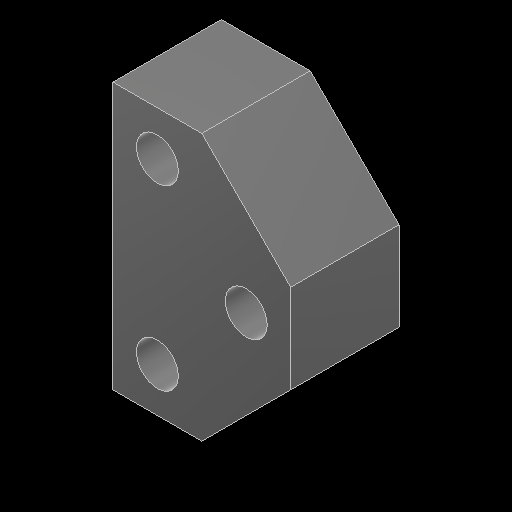
# Autodesk Inventor part: MiddleClampingTopPiece
Saved by Autodesk Inventor 2022 (Build 260153000, 153)
## iProperties
Created: 2022-06-15
Part Number: MiddleClampingTopPiece
Material: Custom TPU
Document SubType Name: Modeling
Designer: tandu
Density: 1.21 g/cm^3
Appearance: Smooth - Black
Mass: 1.40608 g
Surface Area: 10.8835 cm^2
Volume: 1.16205 cm^3
Author: tandu
Autodesk Inventor part; units mm, degrees
ref_plane "YZ Plane" through (0, 0, 0) normal (1, 0, 0) x (0, 1, 0)
ref_plane "XZ Plane" through (0, 0, 0) normal (0, 1, 0) x (-1, 0, 0)
ref_plane "XY Plane" through (0, 0, 0) normal (0, 0, 1) x (1, 0, 0)
sketch "Sketch1" plane through (0, 0, 0) normal (0, 0, 1) x (1, 0, 0)
  line L0 (5.85, -9.525) -> (-6.85, -9.525) projected
  line L1 (5.85, -9.525) -> (5.85, 9.525) projected
  line L2 (-6.85, 9.525) -> (5.85, 9.525) projected
  line L3 (-6.85, 3.175) -> (-6.85, 9.525) projected
  line L4 (-6.85, 3.175) -> (-0.5, 3.175) projected
  line L5 (-0.5, 3.175) -> (-0.5, -3.175) projected
  line L6 (-0.5, -3.175) -> (-6.85, -3.175) projected
  line L7 (-6.85, -9.525) -> (-6.85, -3.175) projected
  circle A0 centre (-3.675, -6.35) radius 1.5 projected
  circle A1 centre (2.675, 0) radius 1.5 projected
  circle A2 centre (-3.675, 6.35) radius 1.5 projected
  line L8 (-6.85, 3.175) -> (-6.85, -3.175)
  line L9 (-0.5, -9.525) -> (5.85, -3.175)
  line L10 (5.85, 3.175) -> (-0.5, 9.525)
  point P0 (0, 0)
  constraints: 6 end point, 2 horizontal alignment, 2 midpoint, 2 point on line, 1 vertical, 1 other
extrude "Extrusion1" add sketch "Sketch1" along normal blind 5.842 contours L0 L7 L6 L5 L4 L3 L2 L10 L1 L9
sketch "Sketch2" plane through (0, 0, 5.842) normal (0, 0, 1) x (1, 0, 0)
  line L0 (-6.85, 3.175) -> (-0.5, 3.175) projected
  line L1 (-0.5, 3.175) -> (-0.5, -3.175) projected
  line L2 (-0.5, -3.175) -> (-6.85, -3.175) projected
  line L3 (-6.85, -3.175) -> (-6.85, -9.525) projected
  line L4 (-6.85, -9.525) -> (-0.5, -9.525) projected
  line L5 (-0.5, -9.525) -> (5.85, -3.175) projected
  line L6 (5.85, -3.175) -> (5.85, 3.175) projected
  line L7 (5.85, 3.175) -> (-0.5, 9.525) projected
  line L8 (-0.5, 9.525) -> (-6.85, 9.525) projected
  line L9 (-6.85, 9.525) -> (-6.85, 3.175) projected
  circle A0 centre (-3.675, -6.35) radius 1.5 projected
  circle A1 centre (2.675, 0) radius 1.5 projected
  circle A2 centre (-3.675, 6.35) radius 1.5 projected
  line L10 (-6.85, 3.175) -> (-0.5, 3.175) projected
  line L11 (-6.85, -3.175) -> (-6.85, 3.175)
  point P0 (0, 0)
  constraints: 2 end point, 1 vertical
extrude "Extrusion2" add sketch "Sketch2" along normal blind 1.905
body "Solid1"
